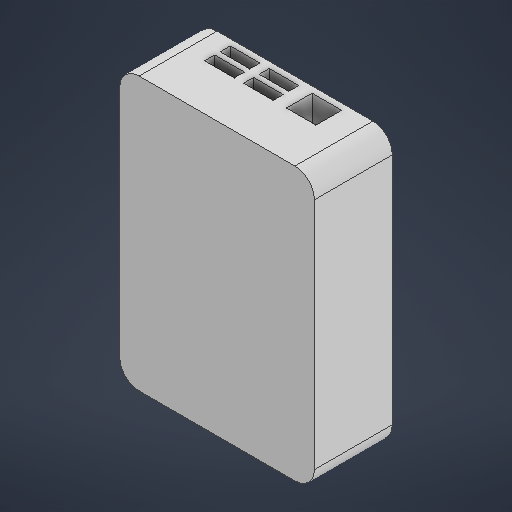
# Autodesk Inventor part: RaspberryPi
Saved by Autodesk Inventor 2026.2 (Build 302298000, 298)
## iProperties
Created: 2026-01-21
Part Number: RaspberryPi
Material: Generic
Document SubType Name: Modeling
Designer: User
Density: 1 g/cm^3
Appearance: Default
Author: User
Autodesk Inventor part; units mm, degrees
ref_plane "YZ Plane" through (0, 0, 0) normal (1, 0, 0) x (0, 1, 0)
ref_plane "XZ Plane" through (0, 0, 0) normal (0, 1, 0) x (-1, 0, 0)
ref_plane "XY Plane" through (0, 0, 0) normal (0, 0, 1) x (1, 0, 0)
sketch "Sketch1" plane through (0, 0, 0) normal (0, 0, 1) x (1, 0, 0)
  line L0 (6.35, 0) -> (57.15, 0)
  line L1 (63.5, 6.35) -> (63.5, 82.55)
  line L2 (57.15, 88.9) -> (6.35, 88.9)
  line L3 (0, 82.55) -> (0, 6.35)
  arc A0 (6.35, 88.9) -> (0, 82.55) centre (6.35, 82.55) ccw
  arc A1 (63.5, 82.55) -> (57.15, 88.9) centre (57.15, 82.55) ccw
  arc A2 (57.15, 0) -> (63.5, 6.35) centre (57.15, 6.35) ccw
  arc A3 (0, 6.35) -> (6.35, 0) centre (6.35, 6.35) ccw
  point P0 (0, 0)
  point P1 (63.5, 88.9)
  point P2 (63.5, 0)
  point P3 (0, 88.9)
  dimension "d0" = 88.9
  dimension "d1" = 63.5
  dimension "d2" = 6.35
  constraints: 8 end point, 8 point on circle, 8 point on line, 8 tangent, 4 centre point, 3 equal radius, 2 parallel, 1 horizontal, 1 perpendicular
  measures "d0" distance of point (63.5, 0) point (63.5, 88.9)
  measures "d1" distance of point (63.5, 88.9) point (0, 88.9)
  measures "d2" radius of A0
extrude "Extrusion1" add sketch "Sketch1" along normal blind 25.4
sketch "Sketch2" plane through (6.35, 88.9, 0) normal (0, 1, 0) x (1, 0, 0)
  line L0 (6.35, -2.032) -> (16.002, -2.032)
  line L1 (16.002, -2.032) -> (16.002, -5.334)
  line L2 (16.002, -5.334) -> (6.35, -5.334)
  line L3 (6.35, -5.334) -> (6.35, -2.032)
  line L4 (0, 0) -> (0, -25.4) projected
  line L5 (50.8, 0) -> (0, 0) projected
  line L6 (28.702, -5.334) -> (19.05, -5.334)
  line L7 (19.05, -2.032) -> (28.702, -2.032)
  line L8 (28.702, -2.032) -> (28.702, -5.334)
  line L9 (19.05, -5.334) -> (19.05, -2.032)
  line L10 (16.002, -10.414) -> (6.35, -10.414)
  line L11 (6.35, -7.112) -> (16.002, -7.112)
  line L12 (16.002, -7.112) -> (16.002, -10.414)
  line L13 (6.35, -10.414) -> (6.35, -7.112)
  line L14 (28.702, -10.414) -> (19.05, -10.414)
  line L15 (19.05, -7.112) -> (28.702, -7.112)
  line L16 (28.702, -7.112) -> (28.702, -10.414)
  line L17 (19.05, -10.414) -> (19.05, -7.112)
  line L18 (33.02, -2.032) -> (42.672, -2.032)
  line L19 (42.672, -2.032) -> (42.672, -10.414)
  line L20 (42.672, -10.414) -> (33.02, -10.414)
  line L21 (33.02, -10.414) -> (33.02, -2.032)
  point P0 (-6.35, 0)
  point P1 (6.35, -3.683)
  point P2 (19.05, -3.683)
  point P3 (6.35, -8.763)
  point P4 (19.05, -8.763)
  point P5 (37.846, -2.032)
  dimension "d5" = 6.35
  dimension "d6" = 9.652
  dimension "d7" = 3.302
  dimension "d8" = 2.032
  dimension "d11" = 12.7
  dimension "d14" = 5.08
  dimension "d17" = 8.382
  dimension "d18" = 9.652
  dimension "d19" = 4.318
  dimension "d20" = 0
  constraints: 40 end point, 4 parallel, 3 horizontal, 2 midpoint, 2 perpendicular, 1 vertical, 27 other
  measures "d5" distance from line of L4 point (6.35, -3.683)
  measures "d6" distance of L0.start L0.end
  measures "d7" distance of L0.end L1.end
  measures "d8" distance between parallel lines of L5 L0
  measures "d11" distance of L1.end L6.start
  measures "d14" distance of L1.end L10.start
  measures "d17" distance of L18.end L19.end
  measures "d18" distance of L18.start L18.end
  measures "d19" distance between parallel lines of L8 L21
  measures "d20" distance from line of point (37.846, -2.032) L7
extrude "Extrusion2" cut sketch "Sketch2" against normal blind 10.16
sketch "Sketch3" plane through (0, 6.35, 0) normal (-1, 0, 0) x (0, 0, 1)
  line L0 (12.7, 10.16) -> (12.7, 15.24) construction
  line L1 (12.065, 10.16) -> (12.065, 15.24)
  line L2 (13.335, 15.24) -> (13.335, 10.16)
  arc A0 (12.065, 10.16) -> (13.335, 10.16) centre (12.7, 10.16) ccw
  arc A1 (13.335, 15.24) -> (12.065, 15.24) centre (12.7, 15.24) ccw
  line L3 (25.4, 76.2) -> (25.4, 0) projected
  line L4 (0, 0) -> (25.4, 0) projected
  line L5 (13.335, 27.94) -> (13.335, 22.86)
  arc A2 (12.065, 22.86) -> (13.335, 22.86) centre (12.7, 22.86) ccw
  line L6 (12.065, 22.86) -> (12.065, 27.94)
  arc A3 (13.335, 27.94) -> (12.065, 27.94) centre (12.7, 27.94) ccw
  line L7 (13.335, 40.64) -> (13.335, 35.56)
  arc A4 (12.065, 35.56) -> (13.335, 35.56) centre (12.7, 35.56) ccw
  line L8 (12.065, 35.56) -> (12.065, 40.64)
  arc A5 (13.335, 40.64) -> (12.065, 40.64) centre (12.7, 40.64) ccw
  circle A6 centre (12.7, 50.8) radius 2.286
  line L9 (0, 76.2) -> (25.4, 76.2) projected
  point P0 (0, -6.35)
  point P1 (12.7, 12.7)
  point P2 (12.7, 76.2)
  dimension "d23" = 5.08
  dimension "d24" = 0.635
  dimension "d25" = 12.7
  dimension "d26" = 12.7
  dimension "d29" = 12.7
  dimension "d34" = 4.572
  dimension "d35" = 12.7
  dimension "d36" = 25.4
  constraints: 16 end point, 12 point on circle, 7 centre point, 4 tangent, 2 midpoint, 2 vertical, 1 parallel, 20 other
  measures "d23" distance of L1.start L1.end
  measures "d24" radius of A1
  measures "d25" distance from line of L3 point (12.7, 12.7)
  measures "d26" distance from line of L4 point (12.7, 12.7)
  measures "d29" distance of L2.start L5.start
  measures "d34" diameter of A6
  measures "d35" distance from line of L3 A6.centre
  measures "d36" distance of point (12.7, 76.2) A6.centre
extrude "Extrusion3" cut sketch "Sketch3" against normal blind 10.16
body "Solid1"
